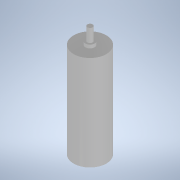
# Autodesk Inventor part: motor
Saved by Autodesk Inventor 2022 (Build 260153000, 153)
## iProperties
Created: 2021-10-06
Part Number: motor
Material: Aluminum 6061
Document SubType Name: Modeling
Designer: Varga Tamás
Density: 2.7 g/cm^3
Appearance: Aluminum - Flat
Mass: 96.6876 g
Surface Area: 68.5653 cm^2
Volume: 35.8102 cm^3
Author: Varga Tamás
Autodesk Inventor part; units mm, degrees
ref_plane "YZ Plane" through (0, 0, 0) normal (1, 0, 0) x (0, 1, 0)
ref_plane "XZ Plane" through (0, 0, 0) normal (0, 1, 0) x (-1, 0, 0)
ref_plane "XY Plane" through (0, 0, 0) normal (0, 0, 1) x (1, 0, 0)
sketch "Sketch1" plane through (0, 0, 0) normal (0, 0, 1) x (1, 0, 0)
  line L0 (0, 0) -> (2, 0)
  line L1 (2, 0) -> (2, -10)
  line L2 (2, -10) -> (3.5, -10)
  line L3 (3.5, -10) -> (3.5, -12.5)
  line L4 (3.5, -12.5) -> (12.5, -12.5)
  line L5 (12.5, -12.5) -> (12.5, -85)
  line L6 (12.5, -85) -> (0, -85)
  line L7 (0, -85) -> (0, 0)
  line L8 (0, -102) -> (0, 17) projected
  dimension "d0" = 2
  dimension "d1" = 3.5
  dimension "d2" = 12.5
  dimension "d3" = 2.5
  dimension "d4" = 12.5
  dimension "d5" = 72.5
  constraints: 16 end point, 7 perpendicular, 1 collinear
  measures "d0" distance of L0.start L0.end
  measures "d1" distance between parallel lines of L7 L3
  measures "d2" distance between parallel lines of L4 L0
  measures "d3" distance of L2.end L3.end
  measures "d4" distance of L5.end L6.end
  measures "d5" distance of L4.end L5.end
revolve "Revolution1" add sketch "Sketch1" angle 360 about axis through (0, -10, 0) along (0, 1, 0)
body "Solid1"
